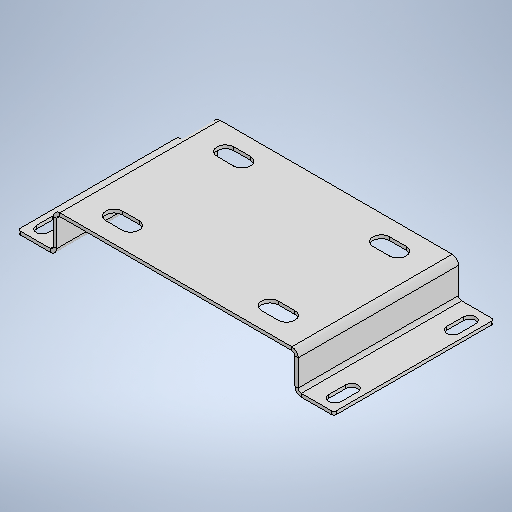
# Autodesk Inventor part: DMF Подставка ркдуктор
Saved by Autodesk Inventor 2026.2 (Build 302298010, 298A)
## iProperties
Created: 2026-06-04
Part Number: DMF Подставка ркдуктор
Material: Stainless Steel
Description: DIE16(5)|\ 90°|corrY -___°|X_____|bom___
Document SubType Name: Sheet Metal
Designer: admin
Stock Number: МОО 305 шпангоут борт
Mass: 1762.25 g
Surface Area: 2283.33 cm^2
Volume: 220.281 cm^3
Density: 8 g/cm^3
Sheet Metal Rule: AISI304 2mm Die16
Sheet Metal Width: 144,000 mm
Sheet Metal Length: 339,573 mm
Sheet Metal Area: 48898,449 mm^2
Appearance: Default
Flat Pattern Width: 14.4 cm
Flat Pattern Length: 33.9573 cm
Flat Pattern Area: 488.984 cm^2
Author: admin
Autodesk Inventor part; units mm, degrees
ref_plane "YZ Plane" through (0, 0, 0) normal (1, 0, 0) x (0, 1, 0)
ref_plane "XZ Plane" through (0, 0, 0) normal (0, 1, 0) x (-1, 0, 0)
ref_plane "XY Plane" through (0, 0, 0) normal (0, 0, 1) x (1, 0, 0)
sketch "Sketch1" plane through (0, 0, 0) normal (0, 0, 1) x (1, 0, 0)
  line L0 (-110, -72) -> (110, -72)
  line L1 (110, -72) -> (110, 72)
  line L2 (110, 72) -> (-110, 72)
  line L3 (-110, 72) -> (-110, -72)
  line L4 (-110, -72) -> (110, 72) construction
  line L5 (110, -72) -> (-110, 72) construction
  circle A0 centre (-70, 50) radius 7.5
  circle A1 centre (-70, -50) radius 7.5
  circle A2 centre (70, 50) radius 7.5
  circle A3 centre (70, -50) radius 7.5
  line L6 (0, 72) -> (0, -72) construction
  line L7 (-110, 0) -> (110, 0) construction
  line L8 (-77.5, 50) -> (-62.5, 50) construction
  line L9 (-77.5, 42.5) -> (-62.5, 42.5)
  line L10 (-62.5, 57.5) -> (-77.5, 57.5)
  arc A4 (-77.5, 57.5) -> (-77.5, 42.5) centre (-77.5, 50) ccw
  arc A5 (-62.5, 42.5) -> (-62.5, 57.5) centre (-62.5, 50) ccw
  arc A6 (77.5, 42.5) -> (77.5, 57.5) centre (77.5, 50) ccw
  line L11 (77.5, 57.5) -> (62.5, 57.5)
  arc A7 (62.5, 57.5) -> (62.5, 42.5) centre (62.5, 50) ccw
  line L12 (62.5, 42.5) -> (77.5, 42.5)
  arc A8 (-62.5, -57.5) -> (-62.5, -42.5) centre (-62.5, -50) ccw
  line L13 (-62.5, -42.5) -> (-77.5, -42.5)
  arc A9 (-77.5, -42.5) -> (-77.5, -57.5) centre (-77.5, -50) ccw
  line L14 (-77.5, -57.5) -> (-62.5, -57.5)
  arc A10 (77.5, -57.5) -> (77.5, -42.5) centre (77.5, -50) ccw
  line L15 (77.5, -42.5) -> (62.5, -42.5)
  arc A11 (62.5, -42.5) -> (62.5, -57.5) centre (62.5, -50) ccw
  line L16 (62.5, -57.5) -> (77.5, -57.5)
  point P0 (0, 0)
  dimension "d154" = 220
  dimension "d155" = 144
  dimension "d157" = 22
  dimension "d158" = 40
  dimension "d159" = 15
  dimension "d160" = 140
  dimension "d161" = 100
  dimension "d190" = 15
  dimension "d193" = 140
  dimension "d196" = 100
  measures "d154" distance of L1.end L2.end
  measures "d155" distance of L0.end L1.end
  measures "d157" distance from line of L2 A0.centre
  measures "d158" distance from line of L3 A0.centre
  measures "d159" diameter of A0
  measures "d160" distance of A2.centre A0.centre
  measures "d161" distance of A3.centre A2.centre
  measures "d190" distance of L8.start L8.end
  measures "d193" distance of L8.end A6.centre
  measures "d196" distance of L8.end A8.centre
extrude "Plate5" add sketch "Sketch1" along normal blind 3
sketch "Sketch7" plane through (-107, 72, 3) normal (-1, 0, 0) x (0, -1, 0)
  line L0 (144, 0) -> (0, 0)
  line L1 (0, 0) -> (0, -35)
  line L2 (0, -35) -> (144, -35)
  line L3 (144, -35) -> (144, 0)
  constraints: 6 end point, 1 horizontal, 1 perpendicular, 1 vertical
edge flange "Flange3" height 35 angle 90 thickness 3 bend radius 2.75 thickness toward (-1, 0, 0) relief round relief width 3 relief depth 1.5 corner gap 2.75 corner form 0 edges at (-110, 0, 0) (110, 0, 0) wall of the first edge with corners at (-107, -72, 3) (-107, 72, 3) (-107, 72, -32) (-107, -72, -32)
bend "Bend3"
corner "Corner3"
sketch "Sketch8" plane through (-107, -72, -29) normal (0, 0, -1) x (-1, 0, 0)
  line L0 (0, 144) -> (0, 0)
  line L1 (0, 0) -> (35, 0)
  line L2 (35, 0) -> (35, 144)
  line L3 (35, 144) -> (0, 144)
  constraints: 6 end point, 1 horizontal, 1 perpendicular, 1 vertical
edge flange "Flange4" height 35 angle 90 thickness 3 bend radius 2.75 thickness toward (0, 0, -1) relief round relief width 3 relief depth 1.5 corner gap 2.75 corner form 0 edges at (-110, 0, -32) (110, 0, -32) wall of the first edge with corners at (-107, 72, -29) (-107, -72, -29) (-142, -72, -29) (-142, 72, -29)
bend "Bend4"
corner "Corner4"
sketch "Sketch9" plane through (-142, -72, -32) normal (0, 0, -1) x (-1, 0, 0)
  line L0 (-10.5, 11.5) -> (-10.5, 26.5) construction
  line L1 (-5, 11.5) -> (-5, 26.5)
  line L2 (-16, 26.5) -> (-16, 11.5)
  arc A0 (-16, 11.5) -> (-5, 11.5) centre (-10.5, 11.5) ccw
  arc A1 (-5, 26.5) -> (-16, 26.5) centre (-10.5, 26.5) ccw
  line L3 (-10.5, 117.5) -> (-10.5, 132.5) construction
  line L4 (-5, 117.5) -> (-5, 132.5)
  line L5 (-16, 132.5) -> (-16, 117.5)
  arc A2 (-16, 117.5) -> (-5, 117.5) centre (-10.5, 117.5) ccw
  arc A3 (-5, 132.5) -> (-16, 132.5) centre (-10.5, 132.5) ccw
  line L6 (0, 144) -> (0, 0) projected
  line L7 (0, 72) -> (-19.5858, 72)
  point P0 (-142, 72)
  point P1 (-10.5, 19)
  point P2 (-10.5, 125)
  point P3 (-10.5, 32)
  point P4 (-10.5, 112)
  dimension "d182" = 11
  dimension "d183" = 15
  dimension "d184" = 5
  dimension "d186" = 80
  constraints: 18 end point, 10 point on circle, 8 tangent, 4 centre point, 3 midpoint, 2 collinear, 2 parallel, 2 vertical, 1 equal radius, 1 horizontal, 1 symmetric about line
  measures "d182" distance between parallel lines of L5 L4
  measures "d183" distance of L3.start L3.end
  measures "d184" distance between parallel lines of L4 L6
  measures "d186" distance of point (-10.5, 32) point (-10.5, 112)
extrude "Cut1" cut sketch "Sketch9" against normal blind 3
mirror "Mirror1" about plane through (0, 0, 0) normal (1, 0, 0) of "Cut1"
fillet "Corner Round2" radius 2 4 edges at (-142, 72, -30.5) (-142, -72, -30.5) (142, -72, -30.5) (142, 72, -30.5)
body "Solid3"
